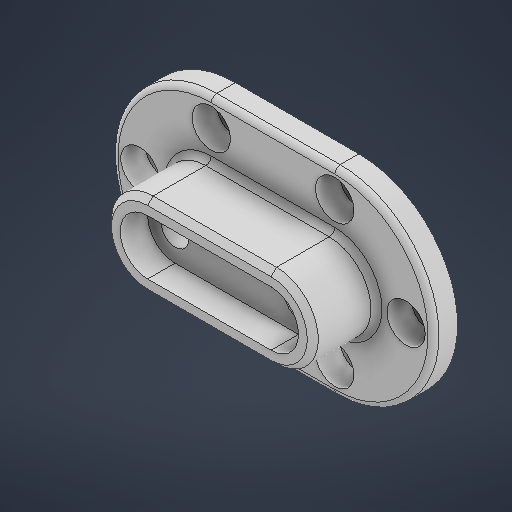
# Autodesk Inventor part: ensayo6
Saved by Autodesk Inventor 2026.2 (Build 302298000, 298)
## iProperties
Created: 2025-12-22
Part Number: ensayo6
Material: Genérico
Document SubType Name: Modeling
Designer: vicho
Density: 1 g/cm^3
Appearance: Valor por defecto
Author: vicho
Autodesk Inventor part; units mm, degrees
ref_plane "YZ Plane" through (0, 0, 0) normal (1, 0, 0) x (0, 1, 0)
ref_plane "XZ Plane" through (0, 0, 0) normal (0, 1, 0) x (-1, 0, 0)
ref_plane "XY Plane" through (0, 0, 0) normal (0, 0, 1) x (1, 0, 0)
sketch "Boceto1" plane through (0, 0, 0) normal (0, 0, 1) x (1, 0, 0)
  line L0 (0, 50) -> (0, -50) construction
  line L1 (-50, 0) -> (50, 0) construction
  circle A0 centre (-11.25, 0) radius 2.5
  circle A1 centre (11.25, 0) radius 2.5
  line L2 (-11.25, 0) -> (11.25, 0) construction
  line L3 (-11.25, -5) -> (11.25, -5)
  line L4 (11.25, 5) -> (-11.25, 5)
  arc A2 (-11.25, 5) -> (-11.25, -5) centre (-11.25, 0) ccw
  arc A3 (11.25, -5) -> (11.25, 5) centre (11.25, 0) ccw
  line L5 (-11.25, 0) -> (11.25, 0) construction
  line L6 (-11.25, -7.6) -> (11.25, -7.6)
  line L7 (11.25, 7.6) -> (-11.25, 7.6)
  arc A4 (-11.25, 7.6) -> (-11.25, -7.6) centre (-11.25, 0) ccw
  arc A5 (11.25, -7.6) -> (11.25, 7.6) centre (11.25, 0) ccw
  line L8 (-11.25, 0) -> (11.25, 0) construction
  line L9 (-11.25, -13) -> (11.25, -13) construction
  line L10 (11.25, 13) -> (-11.25, 13) construction
  arc A6 (-11.25, 13) -> (-11.25, -13) centre (-11.25, 0) ccw construction
  arc A7 (11.25, -13) -> (11.25, 13) centre (11.25, 0) ccw construction
  line L11 (-11.25, 0) -> (11.25, 0) construction
  line L12 (-11.25, -18) -> (11.25, -18)
  line L13 (11.25, 18) -> (-11.25, 18)
  arc A8 (-11.25, 18) -> (-11.25, -18) centre (-11.25, 0) ccw
  arc A9 (11.25, -18) -> (11.25, 18) centre (11.25, 0) ccw
  circle A10 centre (-24.25, 0) radius 1.7
  circle A11 centre (-11.25, -13) radius 1.7
  circle A12 centre (11.25, -13) radius 1.7
  circle A13 centre (24.25, 0) radius 1.7
  circle A14 centre (11.25, 13) radius 1.7
  circle A15 centre (-11.25, 13) radius 1.7
  circle A16 centre (-11.25, 13) radius 3.5
  circle A17 centre (11.25, 13) radius 3.5
  circle A18 centre (24.25, 0) radius 3.5
  circle A19 centre (11.25, -13) radius 3.5
  circle A20 centre (-11.25, -13) radius 3.5
  circle A21 centre (-24.25, 0) radius 3.5
  point P0 (0, 0)
  point P1 (0, 0)
  point P2 (0, 0)
  point P3 (0, 0)
  point P4 (0, 0)
  dimension "d0" = 100
  dimension "d1" = 100
  dimension "d2" = 22.5
  dimension "d3" = 5
  dimension "d4" = 5
  dimension "d5" = 10
  dimension "d6" = 15.2
  dimension "d7" = 26
  dimension "d8" = 36
  dimension "d9" = 18
  dimension "d10" = 31
  dimension "d11" = 3.4
  dimension "d12" = 3.4
  dimension "d13" = 3.4
  dimension "d14" = 3.4
  dimension "d15" = 3.4
  dimension "d16" = 3.4
  dimension "d17" = 7
  dimension "d18" = 7
  dimension "d19" = 7
  dimension "d20" = 7
  dimension "d21" = 7
  dimension "d22" = 7
  constraints: 36 end point, 22 centre point, 19 point on circle, 17 coincident, 16 tangent, 6 midpoint, 4 collinear, 4 parallel, 3 symmetric about line, 2 point on line, 1 horizontal, 1 vertical
  measures "d0" distance of L1.end L1.start
  measures "d1" distance of L0.end L0.start
  measures "d2" distance of point (11.25, 0) point (-11.25, 0)
  measures "d3" diameter of A0
  measures "d4" diameter of A1
  measures "d5" diameter of A3
  measures "d6" diameter of A5
  measures "d7" diameter of A7
  measures "d8" diameter of A9
  measures "d9" distance from line of point (24.25, 0) L13
  measures "d10" distance from line of point (-11.25, -13) L13
  measures "d11" diameter of A10
  measures "d12" diameter of A11
  measures "d13" diameter of A12
  measures "d14" diameter of A13
  measures "d15" diameter of A14
  measures "d16" diameter of A15
  measures "d17" diameter of A16
  measures "d18" diameter of A17
  measures "d19" diameter of A18
  measures "d20" diameter of A19
  measures "d21" diameter of A20
  measures "d22" diameter of A21
extrude "Extrusión1" add sketch "Boceto1" along normal blind 4.4 contours A8 L13 A9 L12
extrude "Extrusión2" add sketch "Boceto1" along normal blind 16 contours A4 L7 A5 L6
extrude "Extrusión3" add sketch "Boceto1" along normal blind 11 contours A2 L4 A3 L3
extrude "Extrusión4" add sketch "Boceto1" against normal blind 1 contours A10 | A12 | A14 | A15 | A16 | A17 | A18 | A19 | A20 | A21
extrude "Extrusión5" cut sketch "Boceto1" against normal blind 4 contours A10 | A12 | A14 | A15
fillet "Empalme1" radius 1 8 edges at (0, -7.6, 4.4) (-18.85, 0, 4.4) (0, 7.6, 4.4) (18.85, 0, 4.4) (0, 18, 4.4) (-29.25, 0, 4.4) (0, -18, 4.4) (29.25, 0, 4.4)
chamfer "Chaflán1" distance 1 angle 45 4 edges at (0, 7.6, 16) (-18.85, 0, 16) (0, -7.6, 16) (18.85, 0, 16)
